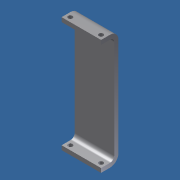
# Autodesk Inventor part: gearbox rib
Saved by Autodesk Inventor 2012 (Build 160160000, 160)
## iProperties
Created: 2012-08-14
Part Number: gearbox rib
Material: Default
Document SubType Name: Sheet Metal
Designer: Bryce
Density: 1 g/cm^3
Sheet Metal Rule: Default
Author: Bryce
Autodesk Inventor part; units mm, degrees
ref_plane "YZ Plane" through (0, 0, 0) normal (1, 0, 0) x (0, 1, 0)
ref_plane "XZ Plane" through (0, 0, 0) normal (0, 1, 0) x (-1, 0, 0)
ref_plane "XY Plane" through (0, 0, 0) normal (0, 0, 1) x (1, 0, 0)
sketch "Sketch1" plane through (0, 0, 0) normal (0, 0, 1) x (1, 0, 0)
  line L0 (-14.2875, 41.656) -> (14.2875, 41.656)
  line L1 (14.2875, 41.656) -> (14.2875, -41.656)
  line L2 (14.2875, -41.656) -> (-14.2875, -41.656)
  line L3 (-14.2875, -41.656) -> (-14.2875, 41.656)
  point P0 (0, 0)
  dimension "d0" = 28.575
  dimension "d1" = 83.312
  dimension "d2" = 14.2875
  dimension "d3" = 41.656
  measures "d0" distance of L0.start L0.end
  measures "d1" distance of L0.end L1.end
  measures "d2" distance from line of point (0, 0) L1
  measures "d3" distance from line of point (0, 0) L2
extrude "Plate2" add sketch "Sketch1" along normal blind 3.048
sketch "Sketch2" plane through (-14.2875, 38.608, 0) normal (0, 1, 0) x (-1, 0, 0)
  line L0 (-28.575, 0) -> (0, 0)
  line L1 (0, 0) -> (0, 12.573)
  line L2 (0, 12.573) -> (-28.575, 12.573)
  line L3 (-28.575, 12.573) -> (-28.575, 0)
  constraints: 4 end point, 4 other
edge flange "Flange1" height 9.525 angle 90 thickness 3.048 bend radius 3.048 thickness toward (0, 1, 0) relief tear relief width 3.048 relief depth 1.524 corner gap 3.048 corner form 0 edges at (0, 41.656, 3.048) (0, -41.656, 3.048) wall of the first edge with corners at (14.2875, 38.608, 0) (-14.2875, 38.608, 0) (-14.2875, 38.608, 12.573) (14.2875, 38.608, 12.573)
bend "Bend1"
corner "Corner1"
sketch "Sketch3" plane through (-14.2875, -38.608, 12.573) normal (0, 1, 0) x (1, 0, 0)
  line L0 (0, 0) -> (0, 6.477) projected
  line L1 (0, 0) -> (28.575, 0) projected
  line L2 (28.575, 0) -> (28.575, 6.477) projected
  point P0 (14.2875, 12.573)
  point P1 (3.175, 3.175)
  point P2 (25.4, 3.175)
  dimension "d16" = 3.175
  dimension "d17" = 3.175
  dimension "d18" = 3.175
  dimension "d19" = 3.175
  measures "d16" distance from line of point (3.175, 3.175) L0
  measures "d17" distance from line of L1 point (3.175, 3.175)
  measures "d18" distance from line of L1 point (25.4, 3.175)
  measures "d19" distance from line of L2 point (25.4, 3.175)
hole "Hole1" at (-11.1125, -38.608, 9.398) at (11.1125, -38.608, 9.398) direction (0, -1, 0) diameter 3.175 end through all
sketch "Sketch5" plane through (-14.2875, 41.656, 12.573) normal (0, 1, 0) x (1, 0, 0)
  circle A0 centre (3.175, 3.175) radius 1.5875 projected
  circle A1 centre (25.4, 3.175) radius 1.5875 projected
  point P0 (14.2875, 12.573)
hole "Hole2" at (-11.1125, 41.656, 9.398) at (11.1125, 41.656, 9.398) direction (0, -1, 0) diameter 3.175 end through all
equation "\"d18\" = d17"
equation "\"d19\" = d16"
equation "\"d25\" = Thickness"
equation "\"d32\" = Thickness"
equation "\"d6\" = BendReliefWidth"
equation "\"d7\" = BendReliefDepth"
equation "\"d8\" = MinimumRemnant"
equation "\"d9\" = BendRadius"
equation "\"d12\" = BendRadius"
equation "\"d13\" = CornerReliefSize"
equation "\"d14\" = GapSize"
equation "\"d15\" = JacobiRadiusSize"
equation "\"d2\" = 0.5 * d0"
equation "\"d3\" = 0.5 * d1"
equation "\"BendRadius\" = Thickness"
equation "\"BendReliefWidth\" = Thickness"
equation "\"BendReliefDepth\" = 0.5 * Thickness"
equation "\"CornerReliefSize\" = 4 * Thickness"
equation "\"MinimumRemnant\" = 2 * Thickness"
equation "\"TransitionRadius\" = BendRadius"
equation "\"JacobiRadiusSize\" = BendRadius"
equation "\"GapSize\" = Thickness"
equation "\"d4\" = BendRadius"
equation "\"d5\" = BendRadius"
equation "\"Thickness\" = 3.048"
body "Solid2"
